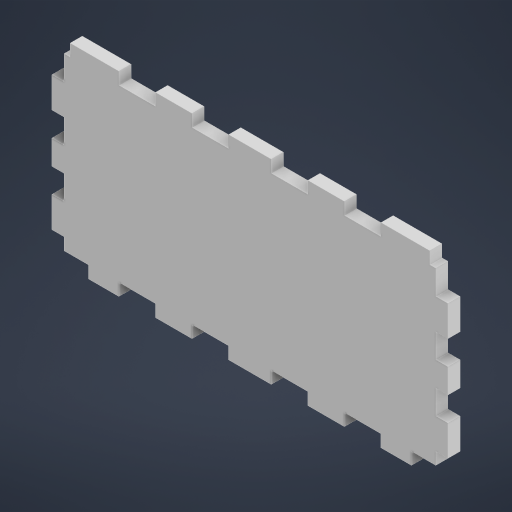
# Autodesk Inventor part: Langbektang houder
Saved by Autodesk Inventor 2023.2 (Build 272271000, 271)
## iProperties
Created: 2020-09-09
Part Number: Langbektang houder
Material: Generic
Document SubType Name: Modeling
Designer: nathan.bollaert
Density: 1 g/cm^3
Appearance: Default
Author: nathan.bollaert
Autodesk Inventor part; units mm, degrees
ref_plane "YZ Plane" through (0, 0, 0) normal (1, 0, 0) x (0, 1, 0)
ref_plane "XZ Plane" through (0, 0, 0) normal (0, 1, 0) x (-1, 0, 0)
ref_plane "XY Plane" through (0, 0, 0) normal (0, 0, 1) x (1, 0, 0)
sketch "Sketch1" plane through (0, 0, 0) normal (0, 0, 1) x (1, 0, 0)
  line L0 (0, -64) -> (130, -64)
  line L1 (130, -64) -> (130, 0)
  line L2 (130, 0) -> (0, 0)
  line L3 (0, 0) -> (0, -64)
  dimension "d228" = 130
  dimension "d229" = 64
  constraints: 8 end point, 2 parallel, 1 coincident, 1 horizontal, 1 perpendicular
  measures "d228" distance of L2.end L1.end
  measures "d229" distance of L1.end L0.end
extrude "Extrusion1" add sketch "Sketch1" against normal blind 4
sketch "Sketch2" plane through (0, 0, 0) normal (0, 0, 1) x (1, 0, 0)
  line L0 (0, -64) -> (0, 0) projected
  line L1 (0, -32) -> (130, -32)
  line L2 (130, 0) -> (130, -64) projected
  line L3 (65, 0) -> (65, -64)
  line L4 (130, -64) -> (0, -64) projected
  line L5 (22, -64) -> (12, -64)
  line L6 (12, -64) -> (12, -60)
  line L7 (22, -60) -> (22, -64)
  line L8 (46, -60) -> (46, -64)
  line L9 (46, -64) -> (34, -64)
  line L10 (34, -64) -> (34, -60)
  line L11 (72, -60) -> (72, -64)
  line L12 (72, -64) -> (58, -64)
  line L13 (58, -64) -> (58, -60)
  line L14 (0, -64) -> (130, -64) projected
  line L15 (96, -64) -> (84, -64)
  line L16 (84, -64) -> (84, -60)
  line L17 (96, -60) -> (96, -64)
  line L18 (118, -60) -> (118, -64)
  line L19 (118, -64) -> (108, -64)
  line L20 (108, -64) -> (108, -60)
  line L21 (0, -46) -> (4, -46)
  line L22 (4, -46) -> (4, -38)
  line L23 (4, -38) -> (0, -38)
  line L24 (0, -38) -> (0, -46)
  line L25 (0, -30) -> (4, -30)
  line L26 (4, -30) -> (4, -22)
  line L27 (4, -22) -> (0, -22)
  line L28 (0, -22) -> (0, -30)
  line L29 (0, 0) -> (0, -64) projected
  line L30 (130, -64) -> (130, 0)
  line L31 (130, 0) -> (130, -64)
  line L32 (0, -60) -> (12, -60)
  line L33 (22, -60) -> (34, -60)
  line L34 (46, -60) -> (58, -60)
  line L35 (72, -60) -> (84, -60)
  line L36 (96, -60) -> (108, -60)
  line L37 (118, -60) -> (130, -60)
  line L38 (0, 0) -> (0, -64)
  line L39 (6, 0) -> (6, -4)
  line L40 (22, -4) -> (22, 0)
  line L41 (46, -4) -> (46, 0)
  line L42 (46, 0) -> (34, 0)
  line L43 (34, 0) -> (34, -4)
  line L44 (72, -4) -> (72, 0)
  line L45 (72, 0) -> (58, 0)
  line L46 (58, 0) -> (58, -4)
  line L47 (96, -4) -> (96, 0)
  line L48 (124, -4) -> (124, 0)
  line L49 (108, 0) -> (108, -4)
  line L50 (96, 0) -> (84, 0)
  line L51 (84, 0) -> (84, -4)
  line L52 (0, -64) -> (0, 0)
  line L53 (130, 0) -> (130, -64)
  line L54 (130, -64) -> (130, 0)
  line L55 (0, -4) -> (6, -4)
  line L56 (22, -4) -> (34, -4)
  line L57 (46, -4) -> (58, -4)
  line L58 (72, -4) -> (84, -4)
  line L59 (96, -4) -> (108, -4)
  line L60 (124, -4) -> (130, -4)
  line L61 (130, -64) -> (130, 0)
  line L62 (130, 0) -> (130, -64)
  line L63 (130, 0) -> (130, -64)
  line L64 (130, -64) -> (130, 0)
  line L65 (0, -60) -> (4, -60)
  line L66 (4, -60) -> (4, -56)
  line L67 (4, -56) -> (0, -56)
  line L68 (0, -56) -> (0, -60)
  line L69 (0, -4) -> (4, -4)
  line L70 (4, -4) -> (4, -12)
  line L71 (4, -12) -> (0, -12)
  line L72 (0, -12) -> (0, -4)
  line L73 (130, -64) -> (130, 0)
  line L74 (130, -46) -> (126, -46)
  line L75 (126, -46) -> (126, -38)
  line L76 (126, -38) -> (130, -38)
  line L77 (130, -38) -> (130, -46)
  line L78 (126, -30) -> (126, -22)
  line L79 (130, -30) -> (126, -30)
  line L80 (126, -22) -> (130, -22)
  line L81 (130, -22) -> (130, -30)
  line L82 (130, 0) -> (130, -64)
  line L83 (130, 0) -> (130, -64)
  line L84 (130, -64) -> (130, 0)
  line L85 (130, -60) -> (126, -60)
  line L86 (126, -60) -> (126, -56)
  line L87 (126, -56) -> (130, -56)
  line L88 (130, -56) -> (130, -60)
  line L89 (130, -4) -> (126, -4)
  line L90 (126, -4) -> (126, -12)
  line L91 (126, -12) -> (130, -12)
  line L92 (130, -12) -> (130, -4)
  line L93 (130, 0) -> (0, 0) projected
  line L94 (130, 0) -> (0, 0)
  point P0 (58, -64)
  point P1 (34, -64)
  point P2 (0, -22)
  point P3 (0, -30)
  point P4 (84, -64)
  point P5 (0, -38)
  point P6 (0, -60)
  point P7 (0, -4)
  point P8 (0, -12)
  point P9 (0, -56)
  point P10 (126, -60)
  point P11 (130, -56)
  point P12 (130, -46)
  point P13 (130, -38)
  point P14 (130, -22)
  point P15 (126, -4)
  point P16 (130, -12)
  dimension "d234" = 10
  dimension "d235" = 12
  dimension "d236" = 12
  dimension "d237" = 12
  dimension "d238" = 14
  dimension "d240" = 12
  dimension "d242" = 12
  dimension "d243" = 10
  dimension "d244" = 12
  dimension "d245" = 12
  dimension "d246" = 12
  dimension "d249" = 8
  dimension "d251" = 8
  dimension "d255" = 8
  dimension "d262" = 4
  dimension "d267" = 8
  dimension "d268" = 10
  dimension "d271" = 10
  dimension "d273" = 6
  dimension "d275" = 12
  constraints: 178 end point, 44 symmetric about line, 32 equal length, 14 point on line, 8 horizontal, 8 perpendicular, 3 midpoint, 1 vertical, 8 other
  measures "d234" distance between parallel lines of L7 L6
  measures "d235" distance between parallel lines of L0 L6
  measures "d236" distance of L8.end L9.end
  measures "d237" distance between parallel lines of L10 L7
  measures "d238" distance of L11.end L12.end
  measures "d240" distance of L8.end L12.end
  measures "d242" distance between parallel lines of L17 L16
  measures "d243" distance of L18.end L19.end
  measures "d244" distance between parallel lines of L20 L17
  measures "d245" distance of L11.end L15.end
  measures "d246" distance of L2.end L18.end
  measures "d249" distance between parallel lines of L23 L21
  measures "d251" distance between parallel lines of L27 L25
  measures "d255" distance between parallel lines of L23 L25
  measures "d262" distance between parallel lines of L4 L32
  measures "d267" distance of L38.end L67.end
  measures "d268" distance of L21.start L67.end
  measures "d271" distance of L27.end L71.end
  measures "d273" distance of L38.start L39.start
  measures "d275" distance of L0.end L71.end
extrude "Extrusion2" cut sketch "Sketch2" against normal blind 4 contours L0 L32 L6 L4 | L0 L67 L66 L32 | L7 L33 L10 L4 | L0 L23 L22 L21 | L8 L34 L13 L4 | L0 L27 L26 L25 | L11 L35 L16 L4 | L0 L55 L70 L71 | L79 L78 L80 L2 | L2 L74 L75 L76 | L93 L51 L58 L44 | L46 L57 L41 L93 | L0 L93 L39 L55 | L17 L36 L20 L4 | L91 L90 L60 L2 | L2 L37 L86 L87 | L93 L49 L59 L47 | L43 L56 L40 L93 | L60 L48 L93 L2 | L2 L4 L18 L37
body "Solid5"
